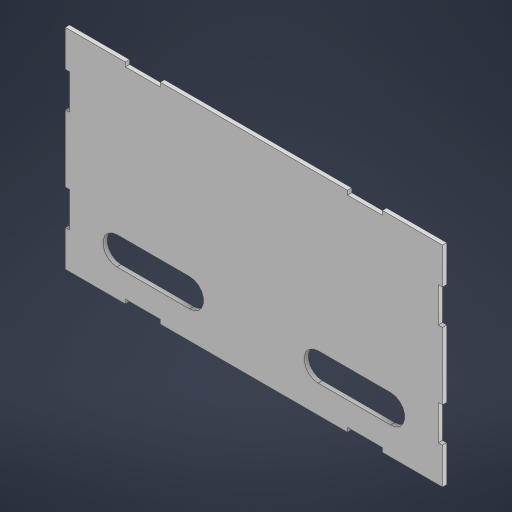
# Autodesk Inventor part: side_part2
Saved by Autodesk Inventor 2023 (Build 270158000, 158)
## iProperties
Created: 2022-11-27
Part Number: side_part2
Material: Generic
Document SubType Name: Modeling
Designer: washington
Density: 1 g/cm^3
Appearance: Default
Author: washington
Autodesk Inventor part; units mm, degrees
ref_plane "YZ Plane" through (0, 0, 0) normal (1, 0, 0) x (0, 1, 0)
ref_plane "XZ Plane" through (0, 0, 0) normal (0, 1, 0) x (-1, 0, 0)
ref_plane "XY Plane" through (0, 0, 0) normal (0, 0, 1) x (1, 0, 0)
sketch "Sketch1" plane through (0, 0, 0) normal (0, 0, 1) x (1, 0, 0)
  line L0 (-135, 75) -> (135, 75)
  line L1 (-135, 75) -> (135, -75) construction
  line L2 (135, 75) -> (-135, -75) construction
  line L3 (-98, -45) -> (-46, -45) construction
  line L4 (-98, -55) -> (-46, -55)
  line L5 (-46, -35) -> (-98, -35)
  arc A0 (-98, -35) -> (-98, -55) centre (-98, -45) ccw
  arc A1 (-46, -55) -> (-46, -35) centre (-46, -45) ccw
  line L6 (46, -45) -> (98, -45) construction
  line L7 (46, -55) -> (98, -55)
  line L8 (98, -35) -> (46, -35)
  arc A2 (46, -35) -> (46, -55) centre (46, -45) ccw
  arc A3 (98, -55) -> (98, -35) centre (98, -45) ccw
  line L9 (135, 49) -> (132, 49)
  line L10 (132, 49) -> (132, 24)
  line L11 (132, 24) -> (135, 24)
  line L12 (135, 75) -> (135, 49)
  line L13 (0, 0) -> (166, 0)
  line L14 (135, -49) -> (132, -49)
  line L15 (132, -49) -> (132, -24)
  line L16 (132, -24) -> (135, -24)
  line L17 (135, 24) -> (135, -24)
  line L18 (135, -49) -> (135, -75)
  line L19 (-135, 49) -> (-132, 49)
  line L20 (-132, 49) -> (-132, 24)
  line L21 (-132, 24) -> (-135, 24)
  line L22 (-135, 49) -> (-135, 75)
  line L23 (-135, -49) -> (-132, -49)
  line L24 (-132, -49) -> (-132, -24)
  line L25 (-132, -24) -> (-135, -24)
  line L26 (-135, -75) -> (-135, -49)
  line L27 (-135, -24) -> (-135, 24)
  line L28 (-92, -75) -> (-92, -72)
  line L29 (-92, -72) -> (-67, -72)
  line L30 (-67, -72) -> (-67, -75)
  line L31 (-92, -75) -> (-135, -75)
  line L32 (0, 0) -> (0, 91)
  line L33 (92, -75) -> (92, -72)
  line L34 (92, -72) -> (67, -72)
  line L35 (67, -72) -> (67, -75)
  line L36 (135, -75) -> (92, -75)
  line L37 (67, -75) -> (-67, -75)
  line L38 (-92, 75) -> (-92, 72)
  line L39 (-92, 72) -> (-67, 72)
  line L40 (-67, 72) -> (-67, 75)
  line L41 (92, 75) -> (92, 72)
  line L42 (92, 72) -> (67, 72)
  line L43 (67, 72) -> (67, 75)
  point P0 (-72, -45)
  point P1 (72, -45)
  dimension "d0" = 270
  dimension "d1" = 150
  dimension "d2" = 37
  dimension "d3" = 37
  dimension "d4" = 52
  dimension "d5" = 52
  dimension "d6" = 30
  dimension "d7" = 10
  dimension "d8" = 10
  dimension "d11" = 3
  dimension "d12" = 25
  dimension "d13" = 26
  dimension "d14" = 0
  dimension "d15" = 31
  dimension "d16" = 25
  dimension "d17" = 26
  dimension "d18" = 3
  dimension "d19" = 267
  dimension "d20" = 25
  dimension "d21" = 3
  dimension "d22" = 43
  dimension "d23" = 124
  dimension "d24" = 42
  constraints: 92 end point, 20 symmetric about line, 14 parallel, 13 perpendicular, 8 point on circle, 8 tangent, 5 horizontal, 4 centre point, 4 midpoint, 2 point on line, 2 vertical
  measures "d0" distance of L1.end L2.end
  measures "d1" distance of L0.end L1.end
  measures "d2" horizontal distance of L3.start L2.end
  measures "d3" horizontal distance of L6.end L1.end
  measures "d4" distance of L3.end L3.start
  measures "d5" distance of L6.end L6.start
  measures "d6" vertical distance of L3.start L2.end
  measures "d7" radius of A0
  measures "d8" radius of A2
  measures "d11" distance of L10.end L11.end
  measures "d12" distance of L9.end L10.end
  measures "d13" distance from line of L0 L9.start
  measures "d14" distance between parallel lines of L17 L12
  measures "d15" distance from line of L13.end L12
  measures "d16" distance of L19.end L20.end
  measures "d17" distance from line of L0 L19.end
  measures "d18" distance of L20.end L21.end
  measures "d19" distance between parallel lines of L20 L18
  measures "d20" distance of L28.end L29.end
  measures "d21" distance of L28.start L28.end
  measures "d22" distance of L2.end L28.start
  measures "d23" distance between parallel lines of L37 L9
  measures "d24" distance from line of L32.end L9
extrude "Extrusion1" add sketch "Sketch1" along normal blind 3 contours L0 L38 L39 L40 L32 L13 L17 L16 L15 L14 L18 L36 L33 L34 L35 L37 L30 L29 L28 L31 L26 L23 L24 L25 L27 L21 L20 L19 L22 | L0 L43 L42 L41 L12 L9 L10 L11 L17 L13 L32
body "Solid1"
